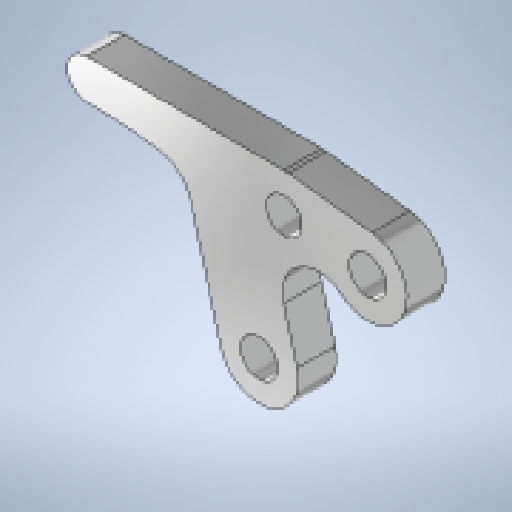
# Autodesk Inventor part: Lever
Saved by Autodesk Inventor 2023.2 (Build 272271000, 271)
## iProperties
Created: 2024-02-17
Part Number: Lever
Material: Aluminum 6061
Document SubType Name: Modeling
Designer: Nathan Cai
Density: 2.7 g/cm^3
Appearance: Aluminum - Flat
Arm_Length: 0.438 in
Arm_Angle: 105.00 deg
Author: Nathan Cai
Autodesk Inventor part; units mm, degrees
ref_plane "YZ Plane" through (0, 0, 0) normal (1, 0, 0) x (0, 1, 0)
ref_plane "XZ Plane" through (0, 0, 0) normal (0, 1, 0) x (-1, 0, 0)
ref_plane "XY Plane" through (0, 0, 0) normal (0, 0, 1) x (1, 0, 0)
sketch "Sketch1" plane through (0, 0, 0) normal (0, 0, 1) x (1, 0, 0)
  circle A0 centre (0, 0) radius 1.4224
  circle A1 centre (0, 0) radius 3.175
  line L0 (0, 0) -> (-15.875, 0) construction
  circle A2 centre (-2.0016, -10.9307) radius 3.175
  circle A3 centre (-2.0016, -10.9307) radius 5 construction
  circle A4 centre (-2.0016, -10.9307) radius 1.5
  line L1 (0, 0) -> (-2.0016, -10.9307) construction
  line L2 (-2.0016, -10.9307) -> (-3.4771, -10.6606) construction
  line L3 (0, 0) -> (-2.0016, -10.9307) construction
  arc A5 (-5.0684, -10.109) -> (1.0652, -11.7525) centre (-2.0016, -10.9307) ccw
  arc A6 (-1.2212, -2.9308) -> (-15.875, 0) centre (-15.875, -38.1) ccw
  arc A7 (-15.875, 3.175) -> (-15.875, 0) centre (-15.875, 1.5875) ccw
  line L4 (-15.875, 3.175) -> (0, 3.175)
  line L5 (-2.0016, -10.9307) -> (-4.9305, 0) construction
  line L6 (1.0652, -10.109) -> (-1.8637, 0.8218)
  line L7 (-7.9973, -0.8218) -> (-5.0684, -11.7525)
  arc A8 (-5.0684, -11.7525) -> (1.0652, -10.109) centre (-2.0016, -10.9307) ccw
  arc A9 (-1.8637, 0.8218) -> (-7.9973, -0.8218) centre (-4.9305, 0) ccw
  circle A10 centre (6.7469, -0.7937) radius 3.175
  circle A11 centre (6.7469, -0.7937) radius 1.5
  line L8 (7.1178, 2.3595) -> (0.371, 3.1533)
  arc A12 (4.6726, -3.1975) -> (-0.0011, -6.1296) centre (2.7869, -5.3826) ccw
  circle A13 centre (6.7469, -0.7937) radius 5 construction
  point P0 (-5.0684, -10.109)
  point P1 (0, 3.175)
  point P2 (-7.9969, -0.8234)
  point P3 (1.0652, -10.109)
  point P4 (-0.8218, -3.0668)
  point P5 (-2.4653, 2.0008)
  point P6 (0.6312, -3.1116)
  point P7 (1.4598, -2.8195)
  point P8 (-1.4243, -1.0642)
  point P9 (-1.7024, 0.5129)
  point P10 (1.0652, -10.109)
  point P11 (-5.0684, -11.7525)
  dimension "d24" = 3
  dimension "d0" = 2.8448
  dimension "d1" = 6.35
  dimension "d9" = 15.875
  dimension "d22" = 6.35
  dimension "d23" = 10
  dimension "Arm_Length" = 11.1125
  dimension "d29" = 3.175
  dimension "d30" = 6.35
  dimension "d31" = 6.35
  dimension "d32" = 3
  dimension "d36" = 10
  dimension "Arm_Angle" = 105
  dimension "d38" = 4.7625
  dimension "d39" = 6.7469
  dimension "d40" = 0.7937
  constraints: 22 end point, 16 point on circle, 14 tangent, 13 centre point, 6 coincident, 2 point on line, 1 concentric, 1 horizontal, 1 parallel, 1 perpendicular, 3 other
  measures "d0" diameter of A0
  measures "d1" diameter of A1
  measures "d9" distance of L0.start L0.end
  measures "d22" diameter of A2
  measures "d23" diameter of A3
  measures "Arm_Length" distance from line of point (0, 0) L2
  measures "d29" diameter of A7
  measures "d30" diameter of A9
  measures "d31" diameter of A10
  measures "d32" diameter of A11
  measures "d36" diameter of A13
  measures "Arm_Angle" angle of L0 L5
  measures "d38" distance from line of A0.centre L5
  measures "d39" horizontal distance of A0.centre A11.centre
  measures "d40" vertical distance of A0.centre A11.centre
extrude "Extrusion1" add sketch "Sketch1" along normal blind 3.048
fillet "Fillet1" radius 3.175 1 edges at (-7.9969, -0.8234, 1.524)
body "Solid1"
